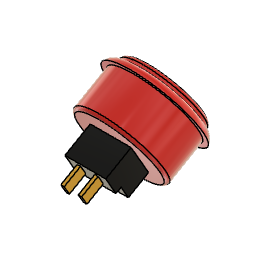
sanwa button v5 (Autodesk Fusion 360 design; units mm, degrees)
Autodesk Fusion 360 part; units mm, degrees
sketch "Sketch1" plane through (0, 0, 0) normal (0, 0, 1) x (1, 0, 0)
  circle A0 centre (0, 0) radius 14.75
  dimension "d1" = 29.5
  constraint coincident A0.centre origin
  measures "d1" diameter of A0
extrude "Extrude1" add sketch "Sketch1" along normal blind 14
sketch "Sketch2" plane through (0, 0, 14) normal (0, 0, 1) x (-1, 0, 0)
  circle A0 centre (0, 0) radius 14.75
  circle A1 centre (0, 0) radius 16.5
  dimension "d4" = 33
  constraint concentric A0 A1
  measures "d4" diameter of A1
extrude "Extrude2" add sketch "Sketch2" along normal blind 2.5 contours A0 | A1
fillet "Fillet1" radius 3 1 edges at (15.3834, 5.9667, 16.5)
sketch "Sketch3" plane through (0, 0, 16.5) normal (0, 0, 1) x (-1, 0, 0)
  circle A0 centre (0, 0) radius 13.542
  circle A1 centre (0, 0) radius 13.542
  constraint concentric A0 A1
extrude "Extrude3" add sketch "Sketch3" along normal blind 2
fillet "Fillet2" radius 1 1 edges at (12.6255, 4.897, 18.5)
sketch "Sketch4" plane through (0, 0, 0) normal (0, 0, -1) x (1, 0, 0)
  circle A0 centre (0, 0) radius 14.75
  line L0 (7, 6) -> (-7, 6)
  line L1 (-7, 6) -> (-7, -6)
  line L2 (-7, -6) -> (7, -6)
  line L3 (7, -6) -> (7, 6)
  line L4 (7, 6) -> (-7, -6) construction
  line L5 (-7, 6) -> (7, -6) construction
  dimension "d13" = 14
  dimension "d14" = 12
  constraint horizontal L0
  constraint perpendicular L0 L1
  constraint parallel L0 L2
  constraint parallel L1 L3
  constraint coincident L4 A0.centre
  constraint coincident L5 A0.centre
  constraint coincident A0.centre origin
  measures "d13" distance of L1.end L2.end
  measures "d14" distance of L0.end L1.end
extrude "Extrude4" add sketch "Sketch4" along normal blind 8 contours L0 L1 L2 L3
sketch "Sketch5" plane through (0, 0, -8) normal (0, 0, -1) x (1, 0, 0)
  line L0 (7, -6) -> (7, 6)
  line L1 (7, 6) -> (-7, 6)
  line L2 (-7, 6) -> (-7, -6)
  line L3 (-7, -6) -> (7, -6)
  line L4 (-7, -6) -> (7, -6)
  line L5 (7, -6) -> (7, 1)
  line L6 (7, 1) -> (-7, 1)
  line L7 (-7, 1) -> (-7, -6)
  dimension "d17" = 7
  constraint horizontal L4
  constraint vertical L5
  constraint horizontal L6
  constraint vertical L7
  constraint coincident L2.end L3.start
  measures "d17" distance of L2.end L6.end
extrude "Extrude5" add sketch "Sketch5" along normal blind 2 contours L0 L2 L3 L4 L5 L6 L7
sketch "Sketch6" plane through (0, 0, -10) normal (0, 0, -1) x (1, 0, 0)
  line L0 (-7, 1) -> (-7, -6)
  line L1 (-7, -6) -> (7, -6)
  line L2 (7, -6) -> (7, 1)
  line L3 (7, 1) -> (-7, 1)
  line L4 (-3.587, -0.8825) -> (-2.4394, -0.8825)
  line L5 (-2.4394, -0.8825) -> (-2.4394, -4.4629)
  line L6 (-2.4394, -4.4629) -> (-3.587, -4.4629)
  line L7 (-3.587, -4.4629) -> (-3.587, -0.8825)
  line L8 (-2.4394, -0.8825) -> (-2.4394, -4.4629)
  line L9 (-3.587, -0.8825) -> (-2.4394, -0.8825)
  line L10 (-3.587, -4.4629) -> (-3.587, -0.8825)
  line L11 (-3.587, -0.8825) -> (-2.4394, -0.8825)
  line L12 (-3.587, -4.4629) -> (-3.587, -0.8825)
  line L13 (-2.4394, -0.8825) -> (-2.4394, -4.4629)
  line L14 (3.5606, -0.8825) -> (3.5606, -4.4629)
  line L15 (2.413, -0.8825) -> (3.5606, -0.8825)
  line L16 (2.413, -4.4629) -> (2.413, -0.8825)
  line L17 (3.5606, -4.4629) -> (2.413, -4.4629)
  constraint horizontal L4
  constraint vertical L5
  constraint horizontal L6
  constraint vertical L7
  constraint horizontal L9
  constraint vertical L8
  constraint vertical L10
  constraint vertical L12
  constraint horizontal L11
  constraint vertical L13
  constraint horizontal L17
  constraint vertical L16
  constraint horizontal L15
  constraint vertical L14
extrude "Extrude6" add sketch "Sketch6" along normal blind 6.5 contours L4 L5 L6 L7 L8 L9 L10 L11 L12 L13 | L14 L15 L16 L17
fillet "Fillet3" radius 1 1 edges at (-13.7518, -5.3338, 0)
move_body "Move1" bodies 1 to x (1, 0, 0) y (0, 0.5, -0.866025) z (0, 0.866025, 0.5) at (0, 11.6603, 0.1962)
move_body "Move2" bodies 1 to x (-1, 0, 0) y (0, 0.5, 0.866025) z (0, 0.866025, -0.5) at (14, -0.3397, 0.5885)
